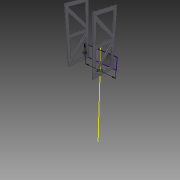
# Autodesk Inventor part: BASE
Saved by Autodesk Inventor 2017 (Build 210142000, 142)
## iProperties
Created: 2017-04-01
Part Number: BASE
Material: Generic
Document SubType Name: Sheet Metal
Designer: Muchen
Density: 1 g/cm^3
Sheet Metal Rule: Default_mm
Appearance: Default
Mass: 141.448 g
Surface Area: 1000.13 cm^2
Volume: 141.448 cm^3
Author: Muchen
Autodesk Inventor part; units mm, degrees
ref_plane "YZ Plane" through (0, 0, 0) normal (1, 0, 0) x (0, 1, 0)
ref_plane "XZ Plane" through (0, 0, 0) normal (0, 1, 0) x (-1, 0, 0)
ref_plane "XY Plane" through (0, 0, 0) normal (0, 0, 1) x (1, 0, 0)
sketch "Sketch1" plane through (0, 0, 0) normal (0, 1, 0) x (-1, 0, 0)
  line L0 (0, 0) -> (180, 0)
  line L1 (180, 0) -> (180, -60)
  line L2 (180, -60) -> (0, -60)
  line L3 (0, -60) -> (0, 0)
  dimension "d0" = 180
  dimension "d34" = 60
  constraints: 8 end point, 2 parallel, 1 horizontal, 1 perpendicular
  measures "d0" distance of L1.end L2.end
  measures "d34" distance of L0.end L1.end
extrude "Plate1" add sketch "Sketch1" along normal blind 3
sketch "Sketch2" plane through (0, 3, 0) normal (0, 1, 0) x (1, 0, 0)
  line L0 (0, 60) -> (0, 0) projected
  line L1 (-180, 0) -> (-180, 60) projected
  line L2 (-133, 18.2) -> (-47, 18.2) construction
  line L3 (-180, 60) -> (0, 60) construction
  circle A0 centre (-103, 147.6372) radius 2 projected
  circle A1 centre (-47, 147.6372) radius 2 projected
  line L4 (-40, 142.6372) -> (-110, 142.6372) projected
  line L5 (-110, 142.6372) -> (-110, 152.6372) projected
  line L6 (-110, 152.6372) -> (-40, 152.6372) projected
  line L7 (-40, 152.6372) -> (-40, 142.6372) projected
  circle A2 centre (-103, 162.6372) radius 2 projected
  circle A3 centre (-47, 162.6372) radius 2 projected
  line L8 (-40, 157.6372) -> (-110, 157.6372) projected
  line L9 (-110, 157.6372) -> (-110, 167.6372) projected
  line L10 (-110, 167.6372) -> (-40, 167.6372) projected
  line L11 (-40, 167.6372) -> (-40, 157.6372) projected
  circle A4 centre (-103, 177.6372) radius 2 projected
  circle A5 centre (-47, 177.6372) radius 2 projected
  line L12 (-110, 182.6372) -> (-40, 182.6372) projected
  line L13 (-40, 182.6372) -> (-40, 172.6372) projected
  line L14 (-40, 172.6372) -> (-110, 172.6372) projected
  line L15 (-110, 172.6372) -> (-110, 182.6372) projected
  circle A6 centre (-103, 192.6372) radius 2 projected
  circle A7 centre (-47, 192.6372) radius 2 projected
  line L16 (-40, 187.6372) -> (-110, 187.6372) projected
  line L17 (-110, 187.6372) -> (-110, 197.6372) projected
  line L18 (-110, 197.6372) -> (-40, 197.6372) projected
  line L19 (-40, 197.6372) -> (-40, 187.6372) projected
  point P0 (-47, 10)
  point P1 (-133, 10)
  point P2 (-90, 18.2)
  point P3 (-90, 60)
  dimension "d4" = 8.2
  dimension "d31" = 86
  dimension "d56" = 10
  constraints: 3 vertical alignment, 2 end point, 2 horizontal alignment, 2 midpoint, 1 horizontal
  measures "d4" distance of point (-47, 10) L2.end
  measures "d31" distance of point (-133, 10) point (-47, 10)
  measures "d56" vertical distance of L0.end point (-47, 10)
hole "Hole1" at (-47, 3, -18.2) at (-47, 3, -10) at (-133, 3, -18.2) at (-133, 3, -10) direction (0, -1, 0) diameter 4 end through all
ref_plane "Work Plane1" through (-90, 0, 0) normal (1, 0, 0) x (0, 0, -1)
sketch "Sketch8" plane through (0, 0, 0) normal (0, -1, 0) x (1, 0, 0)
  line L0 (-180, 0) -> (-180, -60) projected
  line L1 (0, 0) -> (-180, 0) projected
  line L2 (-180, -60) -> (0, -60) projected
  line L3 (0, -60) -> (0, 0) projected
  line L4 (-175, -55) -> (-175, -5) construction
  line L5 (-175, -5) -> (-5, -5) construction
  line L6 (-5, -5) -> (-5, -55) construction
  line L7 (-5, -55) -> (-175, -55) construction
  dimension "d57" = 5
  constraints: 8 end point, 4 coincident, 3 other
  measures "d57" distance between parallel lines of L0 L4
hole "Hole3" at (-175, 0, -5) at (-175, 0, -55) at (-5, 0, -55) at (-5, 0, -5) direction (0, 1, 0) diameter 4 end through all
sketch "Sketch9" plane through (0, 0, -60) normal (0, 0, -1) x (-1, 0, 0)
  line L0 (0, 0) -> (180, 0) projected
  line L1 (163, 0) -> (160, 0)
  line L2 (160, 0) -> (160, -120)
  line L3 (160, -120) -> (163, -120)
  line L4 (163, -120) -> (163, 0)
  line L5 (17, 0) -> (20, 0)
  line L6 (20, 0) -> (20, -120)
  line L7 (20, -120) -> (17, -120)
  line L8 (17, -120) -> (17, 0)
  line L9 (160, -120) -> (20, -120) construction
  point P0 (90, -120)
  point P1 (90, 0)
  dimension "d65" = 3
  dimension "d66" = 140
  dimension "d67" = 120
  constraints: 18 end point, 4 parallel, 3 horizontal, 2 midpoint, 2 perpendicular, 2 point on line, 1 collinear, 1 horizontal alignment, 1 vertical alignment
  measures "d65" distance of L6.end L7.end
  measures "d66" distance between parallel lines of L2 L6
  measures "d67" distance of L7.end L5.start
extrude "Extrusion3" add sketch "Sketch9" against normal blind 260
sketch "Sketch10" plane through (-17, -120, -60) normal (1, 0, 0) x (0, 0, -1)
  line L0 (-15, 15) -> (-15, 105)
  line L1 (-15, 105) -> (-101.675, 105)
  line L2 (-101.675, 105) -> (-15, 15)
  line L3 (-35.825, 15) -> (-122.5, 105)
  line L4 (-122.5, 105) -> (-122.5, 15)
  line L5 (-122.5, 15) -> (-35.825, 15)
  line L6 (-137.5, 15) -> (-137.5, 105)
  line L7 (-137.5, 105) -> (-224.175, 15)
  line L8 (-224.175, 15) -> (-137.5, 15)
  line L9 (-245, 15) -> (-158.325, 105)
  line L10 (-158.325, 105) -> (-245, 105)
  line L11 (-245, 105) -> (-245, 15)
  line L12 (-260, 0) -> (-260, 120) projected
  line L13 (-60, 120) -> (-260, 120) projected
  line L14 (0, 120) -> (0, 0) projected
  line L15 (0, 0) -> (-260, 0) projected
  point P0 (-8, 8)
  point P1 (-252, 8)
  point P2 (-252, 112)
  point P3 (-130, 8)
  point P4 (-130, 0)
  dimension "d70" = 15
  dimension "d71" = 15
  dimension "d72" = 15
  dimension "d73" = 15
  dimension "d74" = 15
  dimension "d75" = 15
  dimension "d77" = 15
  dimension "d80" = 8
  dimension "d81" = 8
  dimension "d82" = 8
  dimension "d83" = 8
  constraints: 25 end point, 6 perpendicular, 5 point on line, 4 horizontal alignment, 2 parallel, 2 vertical alignment, 1 equal length, 1 midpoint, 1 vertical
  measures "d70" distance between parallel lines of L12 L11
  measures "d71" distance between parallel lines of L13 L10
  measures "d72" distance between parallel lines of L14 L0
  measures "d73" distance from line of L14.end L5
  measures "d74" distance between parallel lines of L9 L7
  measures "d75" distance between parallel lines of L2 L3
  measures "d77" distance between parallel lines of L4 L6
  measures "d80" distance from line of L14 point (-8, 8)
  measures "d81" distance from line of L15 point (-8, 8)
  measures "d82" distance from line of L12 point (-252, 8)
  measures "d83" distance from line of L13 point (-252, 112)
extrude "Extrusion4" cut sketch "Sketch10" against normal through all
hole "Hole4" at (-17, -112, -52) at (-17, -112, 192) at (-17, -8, 192) at (-17, -112, 70) direction (-1, 0, 0) diameter 4 end through all
equation "\"d10\" = Thickness"
equation "\"d63\" = Thickness"
equation "\"BendRadius\" = Thickness"
equation "\"BendReliefWidth\" = Thickness"
equation "\"BendReliefDepth\" = 0.5 * Thickness"
equation "\"CornerReliefSize\" = 4 * Thickness"
equation "\"MinimumRemnant\" = 2 * Thickness"
equation "\"TransitionRadius\" = BendRadius"
equation "\"JacobiRadiusSize\" = BendRadius"
equation "\"GapSize\" = Thickness"
equation "\"d2\" = BendRadius"
equation "\"Thickness\" = 3"
body "Solid1"
